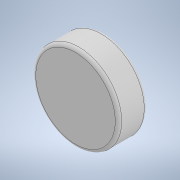
# Autodesk Inventor part: FS-02-SLBV7
Saved by Autodesk Inventor 2022.2 (Build 262287000, 287)
## iProperties
Created: 2021-12-15
Part Number: FS-02-SLBV7
Material: Generic
Document SubType Name: Modeling
Designer: Frank
Density: 1 g/cm^3
Appearance: Default
Author: Frank
Autodesk Inventor part; units mm, degrees
ref_plane "YZ Plane" through (0, 0, 0) normal (1, 0, 0) x (0, 1, 0)
ref_plane "XZ Plane" through (0, 0, 0) normal (0, 1, 0) x (-1, 0, 0)
ref_plane "XY Plane" through (0, 0, 0) normal (0, 0, 1) x (1, 0, 0)
sketch "Sketch1" plane through (0, 0, 0) normal (1, 0, 0) x (0, 1, 0)
  line L0 (4, 1.35) -> (0, 1.35)
  line L1 (0, 1.35) -> (0, -1.35)
  line L2 (0, -1.35) -> (4, -1.35)
  line L3 (4, -1.35) -> (4, 1.35)
  point P0 (0, 0)
  point P1 (0, 0)
  point P2 (4, 0)
  dimension "d0" = 2.7
  dimension "d1" = 8
  constraints: 8 end point, 2 midpoint, 2 parallel, 1 coincident, 1 horizontal, 1 perpendicular
  measures "d0" distance of L0.end L1.end
  measures "d1" diameter of point (4, 0) L1
revolve "Revolution1" add sketch "Sketch1" angle 360 about axis through (0, 0, 1.35) along (0, 0, -1)
fillet "Fillet1" radius 0.3 2 edges at (0, -4, 1.35) (0, -4, -1.35)
body "Solid1"
